Autodesk Fusion 360 part; units mm, degrees
(part 2 of 2)
extrude "Extrude5" cut sketch "ScreenHolder" along normal blind 100 contours A0 | A1 | A2 | A3 | A4 | A5 | A6 | A7 | L17 L18 L19 L20 L23 | L19 L23 L24 L25 L26 bodies 1
extrude "Extrude6" add sketch "PlankTop" along normal blind 4 separate body contours L0 L1 L2 L3 A0 A1 A2 A3 | A4 | A5 | A6 | A7 makes body 2
extrude "Extrude7" cut sketch "Skadis" along normal blind 50 bodies 2
sketch "Sketch14" plane through (0, 0, 0) normal (0, 0, 1) x (1, 0, 0)
extrude "Extrude8" cut sketch "PlankTop" along normal blind 40 keep common part bodies 1
extrude "Extrude9" add sketch "PlankTop" against normal blind 4 separate body makes body 3
extrude "Extrude10" cut sketch "Skadis" against normal blind 120 contours L1 A0 L2 A1 | L26 L27 A25 A26 | L160 L161 A146 A147 | A164 A165 L187 L188 | L195 L196 A174 A175 | L205 L206 A182 A183 bodies 3
move_body "Move1" bodies 3 to x (1, 0, 0) y (0, 1, 0) z (0, 0, 1) at (0, 0, 30)
extrude "Extrude11" cut sketch "ScreenHolder" along normal blind 90 contours L17 L18 L19 L20 L23 | L19 L23 L24 L25 L26 bodies 3
extrude "Extrude12" cut sketch "RaspberryPiDevkKit" along normal blind 100 contours L21 L22 L23 L24 L25 | L29 L30 L31 L32 bodies 3
extrude "Extrude13" add 1 faces at (372.0675, 87.0489, 2.6667) along direction (0, 1, 0) blind 25 on bodies 1 bodies 1
extrude "Extrude14" add 1 faces at (338.4103, 148.2433, 1.3333) along direction (0, 1, 0) blind 55 on bodies 1 bodies 1
extrude "Extrude15" cut 1 faces at (372.0675, 87.0489, 27.3333) along direction (0, 1, 0) blind 30 on bodies 3 bodies 3
fillet "Fillet1" radius 3 4 edges at (378.7342, 117.0489, 28) (358.7342, 117.0489, 28) (358.7342, 87.0489, 28) (378.7342, 87.0489, 28) on bodies 3
fillet "Fillet2" radius 2 4 edges at (334.4103, 203.2433, 28) (346.4103, 203.2433, 28) (346.4103, 148.2433, 28) (334.4103, 148.2433, 28) on bodies 3
fillet "Fillet3" radius 10 8 edges at (179.0201, 107.437, 2) (179.0201, 0, 2) (234.3705, 0, 2) (234.3705, 107.437, 2) (179.0201, 107.437, 28) (179.0201, 0, 28) (234.3705, 0, 28) (234.3705, 107.437, 28) on bodies 1 3
extrude "Extrude16" cut sketch "ScreenHolder" along normal blind 20 contours L32 L33 L34 L35 L39 bodies 1
extrude "Extrude17" cut sketch "ScreenHolder" along normal blind 40 contours A0 | A1 | A2 | A3 bodies 3
extrude "Extrude18" cut sketch "Sketch17" sketch "Sketch19" along normal blind 45 of sketch 2 bodies 3
extrude "Extrude19" cut sketch "Skadis" along normal blind 10 contours L1 A0 L2 A1 | L26 L27 A25 A26 | A164 A165 L187 L188 | L205 L206 A182 A183 bodies 1
extrude "Extrude20" cut sketch "ScreenHolder" along normal blind 11 contours L35 L36 L37 L38 L39 bodies 1
fillet "Fillet4" radius 20 4 edges at (80.5651, 89.3713, 2) (0, 89.3713, 2) (0, 39.3713, 2) (80.5651, 39.3713, 2) on bodies 1
sketch "DownCut" plane through (0, 0, 4) normal (0, 0, 1) x (-1, 0, 0)
  arc A0 (-20, -39.3713) -> (0, -19.3713) centre (-20, -19.3713) ccw
  line L0 (0, -19.3713) -> (0, -10)
  arc A1 (0, -10) -> (-10, 0) centre (-10, -10) ccw
  line L1 (-10, 0) -> (-169.0201, 0)
  arc A2 (-169.0201, 0) -> (-179.0201, -10) centre (-169.0201, -10) ccw
  line L2 (-179.0201, -10) -> (-179.0201, -97.437)
  arc A3 (-189.0201, -107.437) -> (-179.0201, -97.437) centre (-189.0201, -97.437) ccw
  line L3 (-189.0201, -107.437) -> (-224.3705, -107.437)
  arc A4 (-234.3705, -97.437) -> (-224.3705, -107.437) centre (-224.3705, -97.437) ccw
  line L4 (-234.3705, -97.437) -> (-234.3705, -10)
  arc A5 (-234.3705, -10) -> (-244.3705, 0) centre (-244.3705, -10) ccw
  line L5 (-244.3705, 0) -> (-379.754, 0)
  arc A6 (-379.754, 0) -> (-389.754, -10) centre (-379.754, -10) ccw
  line L6 (-389.754, -10) -> (-389.754, -238.8231)
  arc A7 (-389.754, -238.8231) -> (-379.754, -248.8231) centre (-379.754, -238.8231) ccw
  line L7 (-379.754, -248.8231) -> (-10, -248.8231)
  arc A8 (-10, -248.8231) -> (0, -238.8231) centre (-10, -238.8231) ccw
  line L8 (0, -238.8231) -> (0, -109.3713)
  arc A9 (0, -109.3713) -> (-20, -89.3713) centre (-20, -109.3713) ccw
  line L9 (-20, -89.3713) -> (-60.5651, -89.3713)
  arc A10 (-80.5651, -69.3713) -> (-60.5651, -89.3713) centre (-60.5651, -69.3713) ccw
  line L10 (-80.5651, -69.3713) -> (-80.5651, -59.3713)
  arc A11 (-60.5651, -39.3713) -> (-80.5651, -59.3713) centre (-60.5651, -59.3713) ccw
  line L11 (-60.5651, -39.3713) -> (-20, -39.3713)
  line L12 (-371.3372, -216.1319) -> (-371.3372, -231.1319)
  arc A12 (-376.3372, -231.1319) -> (-371.3372, -231.1319) centre (-373.8372, -231.1319) ccw
  line L13 (-376.3372, -231.1319) -> (-376.3372, -216.1319)
  arc A13 (-371.3372, -216.1319) -> (-376.3372, -216.1319) centre (-373.8372, -216.1319) ccw
  line L14 (-371.3372, -16.1319) -> (-371.3372, -31.1319)
  arc A14 (-376.3372, -31.1319) -> (-371.3372, -31.1319) centre (-373.8372, -31.1319) ccw
  line L15 (-376.3372, -31.1319) -> (-376.3372, -16.1319)
  arc A15 (-371.3372, -16.1319) -> (-376.3372, -16.1319) centre (-373.8372, -16.1319) ccw
  arc A16 (-11.3372, -216.1319) -> (-16.3372, -216.1319) centre (-13.8372, -216.1319) ccw
  line L16 (-11.3372, -216.1319) -> (-11.3372, -231.1319)
  arc A17 (-16.3372, -231.1319) -> (-11.3372, -231.1319) centre (-13.8372, -231.1319) ccw
  line L17 (-16.3372, -231.1319) -> (-16.3372, -216.1319)
  line L18 (-11.3372, -16.1319) -> (-11.3372, -31.1319)
  arc A18 (-16.3372, -31.1319) -> (-11.3372, -31.1319) centre (-13.8372, -31.1319) ccw
  line L19 (-16.3372, -31.1319) -> (-16.3372, -16.1319)
  arc A19 (-11.3372, -16.1319) -> (-16.3372, -16.1319) centre (-13.8372, -16.1319) ccw
  circle A20 centre (-379.754, -238.8231) radius 1.5
  circle A21 centre (-10, -10) radius 1.5
  circle A22 centre (-379.754, -10) radius 1.5
  circle A23 centre (-10, -238.8231) radius 1.5
  circle A24 centre (-183.1901, -182.4515) radius 1.7744
  circle A25 centre (-233.3588, -139.2014) radius 1.774
  circle A26 centre (-183.1901, -123.803) radius 1.7744
  circle A27 centre (-233.3588, -167.0532) radius 1.7385
  circle A28 centre (-104.013, -95.4216) radius 1.5
  circle A29 centre (-104.013, -171.9216) radius 1.5
  circle A30 centre (-23.313, -95.4216) radius 1.5
  circle A31 centre (-23.313, -171.9216) radius 1.5
  circle A32 centre (-297.9103, -81.2433) radius 0.85
  circle A33 centre (-366.4103, -203.2433) radius 0.85
  circle A34 centre (-366.4103, -81.2433) radius 0.85
  circle A35 centre (-297.9103, -203.2433) radius 0.85
  circle A36 centre (-256.6953, -107.437) radius 3.15
  circle A37 centre (-169.1953, -19.937) radius 1.55
  circle A38 centre (-156.6953, -7.437) radius 3.15
  circle A39 centre (-244.1953, -94.937) radius 1.55
  circle A40 centre (-256.6953, -7.437) radius 3.15
  circle A41 centre (-169.1953, -94.937) radius 1.55
  circle A42 centre (-156.6953, -107.437) radius 3.15
  circle A43 centre (-244.1953, -19.937) radius 1.55
  circle A44 centre (-10, -10) radius 1.5
  line L20 (0, -238.8231) -> (0, -109.3713)
  line L21 (-10, 0) -> (-169.0201, 0)
  circle A45 centre (-23.313, -95.4216) radius 1.5
  line L22 (-244.3705, 0) -> (-379.754, 0)
  line L23 (-179.0201, -10) -> (-179.0201, -97.437)
  line L24 (-379.754, -248.8231) -> (-10, -248.8231)
  arc A46 (-11.3372, -16.1319) -> (-16.3372, -16.1319) centre (-13.8372, -16.1319) ccw
  circle A47 centre (-23.313, -171.9216) radius 1.5
  arc A48 (-60.5651, -39.3713) -> (-80.5651, -59.3713) centre (-60.5651, -59.3713) ccw
  circle A49 centre (-244.1953, -19.937) radius 1.55
  circle A50 centre (-156.6953, -107.437) radius 3.15
  arc A51 (-16.3372, -31.1319) -> (-11.3372, -31.1319) centre (-13.8372, -31.1319) ccw
  line L25 (-11.3372, -216.1319) -> (-11.3372, -231.1319)
  line L26 (0, -19.3713) -> (0, -10)
  line L27 (-60.5651, -39.3713) -> (-20, -39.3713)
  arc A52 (-20, -39.3713) -> (0, -19.3713) centre (-20, -19.3713) ccw
  circle A53 centre (-244.1953, -94.937) radius 1.55
  circle A54 centre (-169.1953, -94.937) radius 1.55
  circle A55 centre (-256.6953, -7.437) radius 3.15
  line L28 (-20, -89.3713) -> (-60.5651, -89.3713)
  circle A56 centre (-104.013, -171.9216) radius 1.5
  circle A57 centre (-10, -238.8231) radius 1.5
  line L29 (-389.754, -10) -> (-389.754, -238.8231)
  arc A58 (-80.5651, -69.3713) -> (-60.5651, -89.3713) centre (-60.5651, -69.3713) ccw
  circle A59 centre (-104.013, -95.4216) radius 1.5
  line L30 (-234.3705, -97.437) -> (-234.3705, -10)
  arc A60 (0, -109.3713) -> (-20, -89.3713) centre (-20, -109.3713) ccw
  arc A61 (-10, -248.8231) -> (0, -238.8231) centre (-10, -238.8231) ccw
  line L31 (-80.5651, -69.3713) -> (-80.5651, -59.3713)
  circle A62 centre (-366.4103, -81.2433) radius 0.85
  arc A63 (-16.3372, -231.1319) -> (-11.3372, -231.1319) centre (-13.8372, -231.1319) ccw
  line L32 (-11.3372, -16.1319) -> (-11.3372, -31.1319)
  arc A64 (-11.3372, -216.1319) -> (-16.3372, -216.1319) centre (-13.8372, -216.1319) ccw
  arc A65 (0, -10) -> (-10, 0) centre (-10, -10) ccw
  circle A66 centre (-256.6953, -107.437) radius 3.15
  circle A67 centre (-366.4103, -203.2433) radius 0.85
  circle A68 centre (-297.9103, -203.2433) radius 0.85
  line L33 (-16.3372, -31.1319) -> (-16.3372, -16.1319)
  line L34 (-16.3372, -231.1319) -> (-16.3372, -216.1319)
  line L35 (-189.0201, -107.437) -> (-224.3705, -107.437)
  arc A69 (-169.0201, 0) -> (-179.0201, -10) centre (-169.0201, -10) ccw
  circle A70 centre (-156.6953, -7.437) radius 3.15
  line L36 (-376.3372, -231.1319) -> (-376.3372, -216.1319)
  circle A71 centre (-297.9103, -81.2433) radius 0.85
  circle A72 centre (-379.754, -10) radius 1.5
  arc A73 (-371.3372, -16.1319) -> (-376.3372, -16.1319) centre (-373.8372, -16.1319) ccw
  line L37 (-371.3372, -216.1319) -> (-371.3372, -231.1319)
  circle A74 centre (-379.754, -238.8231) radius 1.5
  arc A75 (-234.3705, -10) -> (-244.3705, 0) centre (-244.3705, -10) ccw
  line L38 (-371.3372, -16.1319) -> (-371.3372, -31.1319)
  circle A76 centre (-183.1901, -182.4515) radius 1.7744
  circle A77 centre (-169.1953, -19.937) radius 1.55
  circle A78 centre (-233.3588, -167.0532) radius 1.7385
  arc A79 (-234.3705, -97.437) -> (-224.3705, -107.437) centre (-224.3705, -97.437) ccw
  arc A80 (-189.0201, -107.437) -> (-179.0201, -97.437) centre (-189.0201, -97.437) ccw
  line L39 (-376.3372, -31.1319) -> (-376.3372, -16.1319)
  arc A81 (-379.754, 0) -> (-389.754, -10) centre (-379.754, -10) ccw
  circle A82 centre (-233.3588, -139.2014) radius 1.774
  arc A83 (-371.3372, -216.1319) -> (-376.3372, -216.1319) centre (-373.8372, -216.1319) ccw
  arc A84 (-376.3372, -31.1319) -> (-371.3372, -31.1319) centre (-373.8372, -31.1319) ccw
  arc A85 (-376.3372, -231.1319) -> (-371.3372, -231.1319) centre (-373.8372, -231.1319) ccw
  arc A86 (-389.754, -238.8231) -> (-379.754, -248.8231) centre (-379.754, -238.8231) ccw
  circle A87 centre (-183.1901, -123.803) radius 1.7744
sketch "TopCut" plane through (0, 0, 30) normal (0, 0, 1) x (-1, 0, 0)
  line L0 (-18.663, -174.9637) -> (-110.0633, -174.9637)
  line L1 (-110.0633, -174.9637) -> (-110.0633, -151.1933)
  line L2 (-110.0633, -151.1933) -> (-18.663, -151.1933)
  line L3 (-18.663, -151.1933) -> (-18.663, -174.9637)
  line L4 (-26.6957, -186.645) -> (-26.6957, -231.645)
  line L5 (-26.6957, -231.645) -> (-196.6957, -231.645)
  line L6 (-196.6957, -231.645) -> (-196.6957, -186.645)
  line L7 (-196.6957, -186.645) -> (-26.6957, -186.645)
  line L8 (-18.663, -115.8685) -> (-110.0633, -115.8685)
  line L9 (-110.0633, -115.8685) -> (-110.0633, -93.6879)
  line L10 (-110.0633, -93.6879) -> (-18.663, -93.6879)
  line L11 (-18.663, -93.6879) -> (-18.663, -115.8685)
  circle A0 centre (-244.1953, -94.937) radius 1.55
  circle A1 centre (-244.1953, -19.937) radius 1.55
  circle A2 centre (-169.1953, -94.937) radius 1.55
  circle A3 centre (-169.1953, -19.937) radius 1.55
  arc A4 (-234.3705, -10) -> (-244.3705, 0) centre (-244.3705, -10) ccw
  line L12 (-244.3705, 0) -> (-379.754, 0)
  arc A5 (-379.754, 0) -> (-389.754, -10) centre (-379.754, -10) ccw
  line L13 (-389.754, -10) -> (-389.754, -238.8231)
  arc A6 (-389.754, -238.8231) -> (-379.754, -248.8231) centre (-379.754, -238.8231) ccw
  line L14 (-379.754, -248.8231) -> (-10, -248.8231)
  arc A7 (-10, -248.8231) -> (0, -238.8231) centre (-10, -238.8231) ccw
  line L15 (0, -238.8231) -> (0, -10)
  arc A8 (0, -10) -> (-10, 0) centre (-10, -10) ccw
  line L16 (-10, 0) -> (-169.0201, 0)
  arc A9 (-169.0201, 0) -> (-179.0201, -10) centre (-169.0201, -10) ccw
  line L17 (-179.0201, -10) -> (-179.0201, -97.437)
  arc A10 (-189.0201, -107.437) -> (-179.0201, -97.437) centre (-189.0201, -97.437) ccw
  line L18 (-189.0201, -107.437) -> (-224.3705, -107.437)
  arc A11 (-234.3705, -97.437) -> (-224.3705, -107.437) centre (-224.3705, -97.437) ccw
  line L19 (-234.3705, -97.437) -> (-234.3705, -10)
  line L20 (-378.7342, -114.0489) -> (-378.7342, -90.0489)
  arc A12 (-375.7342, -87.0489) -> (-378.7342, -90.0489) centre (-375.7342, -90.0489) ccw
  line L21 (-375.7342, -87.0489) -> (-361.7342, -87.0489)
  arc A13 (-358.7342, -90.0489) -> (-361.7342, -87.0489) centre (-361.7342, -90.0489) ccw
  line L22 (-358.7342, -90.0489) -> (-358.7342, -114.0489)
  arc A14 (-361.7342, -117.0489) -> (-358.7342, -114.0489) centre (-361.7342, -114.0489) ccw
  line L23 (-361.7342, -117.0489) -> (-375.7342, -117.0489)
  arc A15 (-378.7342, -114.0489) -> (-375.7342, -117.0489) centre (-375.7342, -114.0489) ccw
  line L24 (-346.4103, -201.2433) -> (-346.4103, -150.2433)
  arc A16 (-344.4103, -148.2433) -> (-346.4103, -150.2433) centre (-344.4103, -150.2433) ccw
  line L25 (-344.4103, -148.2433) -> (-336.4103, -148.2433)
  arc A17 (-334.4103, -150.2433) -> (-336.4103, -148.2433) centre (-336.4103, -150.2433) ccw
  line L26 (-334.4103, -150.2433) -> (-334.4103, -201.2433)
  arc A18 (-336.4103, -203.2433) -> (-334.4103, -201.2433) centre (-336.4103, -201.2433) ccw
  line L27 (-336.4103, -203.2433) -> (-344.4103, -203.2433)
  arc A19 (-346.4103, -201.2433) -> (-344.4103, -203.2433) centre (-344.4103, -201.2433) ccw
  circle A20 centre (-379.754, -10) radius 1.5
  circle A21 centre (-10, -238.8231) radius 1.5
  circle A22 centre (-379.754, -238.8231) radius 1.5
  circle A23 centre (-10, -10) radius 1.5
  line L28 (-216.3372, -231.1319) -> (-216.3372, -216.1319)
  arc A24 (-211.3372, -216.1319) -> (-216.3372, -216.1319) centre (-213.8372, -216.1319) ccw
  line L29 (-211.3372, -216.1319) -> (-211.3372, -231.1319)
  arc A25 (-216.3372, -231.1319) -> (-211.3372, -231.1319) centre (-213.8372, -231.1319) ccw
  arc A26 (-16.3372, -231.1319) -> (-11.3372, -231.1319) centre (-13.8372, -231.1319) ccw
  line L30 (-16.3372, -231.1319) -> (-16.3372, -216.1319)
  arc A27 (-11.3372, -216.1319) -> (-16.3372, -216.1319) centre (-13.8372, -216.1319) ccw
  line L31 (-11.3372, -216.1319) -> (-11.3372, -231.1319)
  line L32 (-376.3372, -231.1319) -> (-376.3372, -216.1319)
  arc A28 (-371.3372, -216.1319) -> (-376.3372, -216.1319) centre (-373.8372, -216.1319) ccw
  line L33 (-371.3372, -216.1319) -> (-371.3372, -231.1319)
  arc A29 (-376.3372, -231.1319) -> (-371.3372, -231.1319) centre (-373.8372, -231.1319) ccw
  line L34 (-216.3372, -191.1319) -> (-216.3372, -176.1319)
  arc A30 (-211.3372, -176.1319) -> (-216.3372, -176.1319) centre (-213.8372, -176.1319) ccw
  line L35 (-211.3372, -176.1319) -> (-211.3372, -191.1319)
  arc A31 (-216.3372, -191.1319) -> (-211.3372, -191.1319) centre (-213.8372, -191.1319) ccw
  line L36 (-16.3372, -31.1319) -> (-16.3372, -16.1319)
  arc A32 (-11.3372, -16.1319) -> (-16.3372, -16.1319) centre (-13.8372, -16.1319) ccw
  line L37 (-11.3372, -16.1319) -> (-11.3372, -31.1319)
  arc A33 (-16.3372, -31.1319) -> (-11.3372, -31.1319) centre (-13.8372, -31.1319) ccw
  line L38 (-376.3372, -31.1319) -> (-376.3372, -16.1319)
  arc A34 (-371.3372, -16.1319) -> (-376.3372, -16.1319) centre (-373.8372, -16.1319) ccw
  line L39 (-371.3372, -16.1319) -> (-371.3372, -31.1319)
  arc A35 (-376.3372, -31.1319) -> (-371.3372, -31.1319) centre (-373.8372, -31.1319) ccw
  circle A36 centre (-10, -10) radius 1.5
  circle A37 centre (-169.1953, -19.937) radius 1.55
  arc A38 (-11.3372, -16.1319) -> (-16.3372, -16.1319) centre (-13.8372, -16.1319) ccw
  arc A39 (-16.3372, -31.1319) -> (-11.3372, -31.1319) centre (-13.8372, -31.1319) ccw
  line L40 (-371.3372, -16.1319) -> (-371.3372, -31.1319)
  line L41 (-16.3372, -231.1319) -> (-16.3372, -216.1319)
  line L42 (-110.0633, -115.8685) -> (-110.0633, -93.6879)
  line L43 (-379.754, -248.8231) -> (-10, -248.8231)
  line L44 (-216.3372, -231.1319) -> (-216.3372, -216.1319)
  line L45 (-389.754, -10) -> (-389.754, -238.8231)
  line L46 (-211.3372, -216.1319) -> (-211.3372, -231.1319)
  line L47 (-110.0633, -174.9637) -> (-110.0633, -151.1933)
  line L48 (-244.3705, 0) -> (-379.754, 0)
  line L49 (-196.6957, -231.645) -> (-196.6957, -186.645)
  line L50 (-216.3372, -191.1319) -> (-216.3372, -176.1319)
  line L51 (-346.4103, -201.2433) -> (-346.4103, -150.2433)
  line L52 (-234.3705, -97.437) -> (-234.3705, -10)
  arc A40 (-10, -248.8231) -> (0, -238.8231) centre (-10, -238.8231) ccw
  line L53 (-110.0633, -93.6879) -> (-18.663, -93.6879)
  line L54 (-361.7342, -117.0489) -> (-375.7342, -117.0489)
  arc A41 (-376.3372, -31.1319) -> (-371.3372, -31.1319) centre (-373.8372, -31.1319) ccw
  arc A42 (-189.0201, -107.437) -> (-179.0201, -97.437) centre (-189.0201, -97.437) ccw
  line L55 (-189.0201, -107.437) -> (-224.3705, -107.437)
  circle A43 centre (-10, -238.8231) radius 1.5
  line L56 (-358.7342, -90.0489) -> (-358.7342, -114.0489)
  arc A44 (-234.3705, -97.437) -> (-224.3705, -107.437) centre (-224.3705, -97.437) ccw
  line L57 (0, -238.8231) -> (0, -10)
  arc A45 (-211.3372, -176.1319) -> (-216.3372, -176.1319) centre (-213.8372, -176.1319) ccw
  arc A46 (-234.3705, -10) -> (-244.3705, 0) centre (-244.3705, -10) ccw
  arc A47 (-216.3372, -231.1319) -> (-211.3372, -231.1319) centre (-213.8372, -231.1319) ccw
  arc A48 (-211.3372, -216.1319) -> (-216.3372, -216.1319) centre (-213.8372, -216.1319) ccw
  line L58 (-211.3372, -176.1319) -> (-211.3372, -191.1319)
  circle A49 centre (-379.754, -10) radius 1.5
  line L59 (-179.0201, -10) -> (-179.0201, -97.437)
  line L60 (-371.3372, -216.1319) -> (-371.3372, -231.1319)
  line L61 (-26.6957, -186.645) -> (-26.6957, -231.645)
  arc A50 (-379.754, 0) -> (-389.754, -10) centre (-379.754, -10) ccw
  line L62 (-10, 0) -> (-169.0201, 0)
  arc A51 (-346.4103, -201.2433) -> (-344.4103, -203.2433) centre (-344.4103, -201.2433) ccw
  line L63 (-334.4103, -150.2433) -> (-334.4103, -201.2433)
  arc A52 (-334.4103, -150.2433) -> (-336.4103, -148.2433) centre (-336.4103, -150.2433) ccw
  line L64 (-375.7342, -87.0489) -> (-361.7342, -87.0489)
  line L65 (-344.4103, -148.2433) -> (-336.4103, -148.2433)
  circle A53 centre (-169.1953, -94.937) radius 1.55
  arc A54 (-336.4103, -203.2433) -> (-334.4103, -201.2433) centre (-336.4103, -201.2433) ccw
  arc A55 (-371.3372, -16.1319) -> (-376.3372, -16.1319) centre (-373.8372, -16.1319) ccw
  line L66 (-196.6957, -186.645) -> (-26.6957, -186.645)
  line L67 (-110.0633, -151.1933) -> (-18.663, -151.1933)
  arc A56 (-16.3372, -231.1319) -> (-11.3372, -231.1319) centre (-13.8372, -231.1319) ccw
  line L68 (-378.7342, -114.0489) -> (-378.7342, -90.0489)
  line L69 (-18.663, -115.8685) -> (-110.0633, -115.8685)
  arc A57 (-389.754, -238.8231) -> (-379.754, -248.8231) centre (-379.754, -238.8231) ccw
  line L70 (-26.6957, -231.645) -> (-196.6957, -231.645)
  circle A58 centre (-379.754, -238.8231) radius 1.5
  arc A59 (-11.3372, -216.1319) -> (-16.3372, -216.1319) centre (-13.8372, -216.1319) ccw
  arc A60 (0, -10) -> (-10, 0) centre (-10, -10) ccw
  line L71 (-11.3372, -16.1319) -> (-11.3372, -31.1319)
  line L72 (-16.3372, -31.1319) -> (-16.3372, -16.1319)
  line L73 (-376.3372, -231.1319) -> (-376.3372, -216.1319)
  line L74 (-336.4103, -203.2433) -> (-344.4103, -203.2433)
  line L75 (-18.663, -151.1933) -> (-18.663, -174.9637)
  line L76 (-11.3372, -216.1319) -> (-11.3372, -231.1319)
  line L77 (-376.3372, -31.1319) -> (-376.3372, -16.1319)
  arc A61 (-169.0201, 0) -> (-179.0201, -10) centre (-169.0201, -10) ccw
  arc A62 (-344.4103, -148.2433) -> (-346.4103, -150.2433) centre (-344.4103, -150.2433) ccw
  line L78 (-18.663, -93.6879) -> (-18.663, -115.8685)
  arc A63 (-358.7342, -90.0489) -> (-361.7342, -87.0489) centre (-361.7342, -90.0489) ccw
  arc A64 (-361.7342, -117.0489) -> (-358.7342, -114.0489) centre (-361.7342, -114.0489) ccw
  arc A65 (-371.3372, -216.1319) -> (-376.3372, -216.1319) centre (-373.8372, -216.1319) ccw
  circle A66 centre (-244.1953, -94.937) radius 1.55
  arc A67 (-375.7342, -87.0489) -> (-378.7342, -90.0489) centre (-375.7342, -90.0489) ccw
  arc A68 (-378.7342, -114.0489) -> (-375.7342, -117.0489) centre (-375.7342, -114.0489) ccw
  circle A69 centre (-244.1953, -19.937) radius 1.55
  line L79 (-18.663, -174.9637) -> (-110.0633, -174.9637)
  arc A70 (-376.3372, -231.1319) -> (-371.3372, -231.1319) centre (-373.8372, -231.1319) ccw
  arc A71 (-216.3372, -191.1319) -> (-211.3372, -191.1319) centre (-213.8372, -191.1319) ccw
move_body "Move2" bodies 2 to x (1, 0, 0) y (0, 1, 0) z (0, 0, 1) at (0, 0, 90)
named bodies: "SkadisHoles", "HolderBody", "TopBody"
